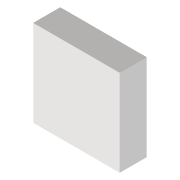
# Autodesk Inventor part: 00_Bluraymirror_6.4x6.4x2mm
Saved by Autodesk Inventor 2022 (Build 260153000, 153)
## iProperties
Created: 2022-04-18
Part Number: 00_Bluraymirror_6.4x6.4x2mm
Material: Generic
Document SubType Name: Modeling
Designer: Prakash Lab
Density: 1 g/cm^3
Appearance: Default
Author: Prakash Lab
Autodesk Inventor part; units mm, degrees
ref_plane "YZ Plane" through (0, 0, 0) normal (1, 0, 0) x (0, 1, 0)
ref_plane "XZ Plane" through (0, 0, 0) normal (0, 1, 0) x (-1, 0, 0)
ref_plane "XY Plane" through (0, 0, 0) normal (0, 0, 1) x (1, 0, 0)
sketch "Sketch1" plane through (0, 0, 0) normal (0, 0, 1) x (1, 0, 0)
  line L0 (3.2, -3.2) -> (-3.2, -3.2)
  line L1 (-3.2, -3.2) -> (-3.2, 3.2)
  line L2 (-3.2, 3.2) -> (3.2, 3.2)
  line L3 (3.2, 3.2) -> (3.2, -3.2)
  line L4 (3.2, -3.2) -> (-3.2, 3.2) construction
  line L5 (-3.2, -3.2) -> (3.2, 3.2) construction
  point P0 (0, 0)
  dimension "d0" = 6.4
  dimension "d1" = 6.4
  constraints: 12 end point, 2 midpoint, 2 parallel, 1 horizontal, 1 perpendicular
  measures "d0" distance of L1.end L2.end
  measures "d1" distance of L0.end L1.end
extrude "Extrusion1" add sketch "Sketch1" along normal blind 2
body "Solid1"
